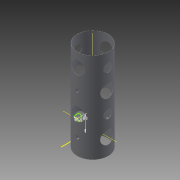
# Autodesk Inventor part: Probe Region Shield
Saved by Autodesk Inventor 2015 (Build 190159000, 159)
## iProperties
Created: 2014-06-23
Part Number: Probe Region Shield
Material: Generic
Document SubType Name: Modeling
Designer: Aki
Density: 1 g/cm^3
Appearance: Default
Author: Aki
Autodesk Inventor part; units mm, degrees
sketch "Sketch1" plane through (0, 0, 0) normal (0, 1, 0) x (-1, 0, 0)
  circle A0 centre (0, 0) radius 82
  circle A1 centre (0, 0) radius 83
  dimension "d0" = 164
  dimension "d1" = 166
  constraints: 2 centre point, 2 coincident
  measures "d0" diameter of A0
  measures "d1" diameter of A1
extrude "Extrusion1" add sketch "Sketch1" along normal blind 466.5 and the other way blind 16
ref_plane "Work Plane1" through (85.5, 0, 0) normal (1, 0, 0) x (0, 1, 0)
ref_plane "Work Plane2" through (-85.5, 0, 0) normal (1, 0, 0) x (0, 1, 0)
sketch "Sketch2" plane through (85.5, 0, 0) normal (1, 0, 0) x (0, 1, 0)
  circle A0 centre (394.5, 0) radius 23.25
  line L0 (466.5, -83) -> (466.5, 83) projected
  line L1 (-16, 83) -> (-16, -83) projected
  point P0 (0, 0)
  dimension "d9" = 46.5
  dimension "d12" = 72
  constraints: 1 centre point, 1 other
  measures "d9" diameter of A0
  measures "d12" distance from line of L0 A0.centre
hole "Hole1" at (85.5, 394.5, 0) direction (-1, 0, 0) diameter 46.5 end through all
sketch "Sketch5" plane through (85.5, 0, 0) normal (1, 0, 0) x (0, 1, 0)
  circle A0 centre (287, 0) radius 35.25
  line L0 (-16, 83) -> (-16, -83) projected
  point P0 (0, 0)
  dimension "d39" = 70.5
  dimension "d62" = 287
  constraints: 1 centre point, 1 other
  measures "d39" diameter of A0
  measures "d62" distance of A0.centre point (0, 0)
hole "Hole4" at (85.5, 287, 0) direction (-1, 0, 0) diameter 70.5 end through all
sketch "Sketch4" plane through (85.5, 0, 0) normal (1, 0, 0) x (0, 1, 0)
  circle A0 centre (179.5, 0) radius 23.25
  line L0 (-16, 83) -> (-16, -83) projected
  point P0 (0, 0)
  dimension "d30" = 46.5
  dimension "d61" = 179.5
  constraints: 1 centre point, 1 other
  measures "d30" diameter of A0
  measures "d61" distance of A0.centre point (0, 0)
hole "Hole3" at (85.5, 179.5, 0) direction (-1, 0, 0) diameter 46.5 end through all
sketch "Sketch3" plane through (85.5, 0, 0) normal (1, 0, 0) x (0, 1, 0)
  circle A0 centre (72, 0) radius 35.25
  line L0 (-16, 83) -> (-16, -83) projected
  point P0 (0, 0)
  dimension "d21" = 70.5
  dimension "d60" = 72
  constraints: 1 centre point, 1 other
  measures "d21" diameter of A0
  measures "d60" distance of A0.centre point (0, 0)
hole "Hole2" at (85.5, 72, 0) direction (-1, 0, 0) diameter 70.5 end through all
ref_plane "Work Plane4" through (0, 0, -85.5) normal (0, 0, 1) x (1, 0, 0)
sketch "Sketch9" plane through (0, 0, -85.5) normal (0, 0, 1) x (1, 0, 0)
  circle A0 centre (0, 394.5) radius 35.25
  line L0 (83, 466.5) -> (-83, 466.5) projected
  point P0 (0, 0)
  dimension "d65" = 70.5
  dimension "d68" = 72
  constraints: 1 centre point
  measures "d65" diameter of A0
  measures "d68" distance from line of L0 A0.centre
sketch "Sketch11" plane through (0, 0, -85.5) normal (0, 0, 1) x (1, 0, 0)
  circle A0 centre (0, 179.5) radius 35.25
  line L0 (83, 466.5) -> (-83, 466.5) projected
  point P0 (0, 0)
  dimension "d69" = 70.5
  dimension "d70" = 287
  constraints: 1 centre point
  measures "d69" diameter of A0
  measures "d70" distance from line of L0 A0.centre
sketch "Sketch12" plane through (0, 0, -85.5) normal (0, 0, 1) x (1, 0, 0)
  circle A0 centre (0, 287) radius 9.9
  line L0 (83, 466.5) -> (-83, 466.5) projected
  point P0 (0, 0)
  dimension "d71" = 19.8
  dimension "d72" = 179.5
  constraints: 1 centre point
  measures "d71" diameter of A0
  measures "d72" distance from line of L0 A0.centre
sketch "Sketch13" plane through (0, 0, -85.5) normal (0, 0, 1) x (1, 0, 0)
  circle A0 centre (0, 72) radius 9.9
  line L0 (83, 466.5) -> (-83, 466.5) projected
  point P0 (0, 0)
  dimension "d73" = 19.8
  dimension "d74" = 394.5
  constraints: 1 centre point
  measures "d73" diameter of A0
  measures "d74" distance from line of L0 A0.centre
hole "Hole5" at (0, 394.5, -85.5) direction (0, 0, 1) diameter 70.5 end through all
hole "Hole6" at (0, 179.5, -85.5) direction (0, 0, 1) diameter 70.5 end through all
hole "Hole7" at (0, 287, -85.5) direction (0, 0, 1) diameter 19.8 end through all
hole "Hole8" at (0, 72, -85.5) direction (0, 0, 1) diameter 19.8 end through all
ref_plane "Work Plane5" through (0, 29.7, 0) normal (0, 1, 0) x (-1, 0, 0)
ref_plane "Work Plane6" through (0, 435, 0) normal (0, 1, 0) x (-1, 0, 0)
sketch "Sketch35" plane through (-85.5, 0, 0) normal (1, 0, 0) x (0, 1, 0)
  circle A0 centre (72, 0) radius 23.25
  line L0 (-16, 83) -> (-16, -83) projected
  point P0 (0, 0)
  dimension "d358" = 46.5
  dimension "d359" = 88
  constraints: 1 centre point
  measures "d358" diameter of A0
  measures "d359" distance from line of L0 A0.centre
body "Solid1"
